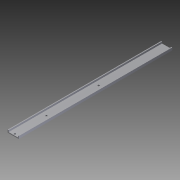
# Autodesk Inventor part: 2
Saved by Autodesk Inventor 2011 (Build 150239000, 239)
## iProperties
Created: 2011-09-24
Part Number: 2
Document SubType Name: Modeling
Designer: Matthew
Density: 1 g/cm^3
Author: Matthew
Autodesk Inventor part; units mm, degrees
ref_plane "YZ Plane" through (0, 0, 0) normal (1, 0, 0) x (0, 1, 0)
ref_plane "XZ Plane" through (0, 0, 0) normal (0, 1, 0) x (-1, 0, 0)
ref_plane "XY Plane" through (0, 0, 0) normal (0, 0, 1) x (1, 0, 0)
sketch "Sketch1" plane through (0, 0, 0) normal (0, 0, 1) x (1, 0, 0)
  line L0 (-18.7296, 9.1612) -> (16.5704, 9.1612)
  line L1 (16.5704, 9.1612) -> (16.5704, -0.3388)
  line L2 (16.5704, -0.3388) -> (-18.7296, -0.3388)
  line L3 (-18.7296, -0.3388) -> (-18.7296, 9.1612)
  line L4 (-18.7296, 4.4112) -> (16.5704, 4.4112)
  line L5 (-18.7296, 4.4112) -> (-18.7296, -0.3388)
  line L6 (-18.7296, 2.0362) -> (16.5704, 2.0362)
  line L7 (16.5704, 4.4112) -> (14.1954, 2.0362)
  line L8 (16.5704, 4.4112) -> (19.9291, 4.4112) construction
  line L9 (-18.7296, 4.4112) -> (-16.3546, 2.0362)
  line L10 (-16.3546, 2.0362) -> (-16.3546, 9.1612)
  line L11 (14.1954, 2.0362) -> (14.1954, 9.1612)
  line L12 (-16.3546, 4.4112) -> (-13.9796, 2.0362)
  line L13 (14.1954, 4.4112) -> (11.8204, 2.0362)
  line L14 (11.8204, 2.0362) -> (11.8204, 9.1612)
  line L15 (-13.9796, 2.0362) -> (-13.9796, 9.1612)
  point P0 (0, 0)
  dimension "d0" = 35.3
  dimension "d1" = 9.5
  dimension "d2" = 135
  constraints: 32 end point, 13 point on line, 8 perpendicular, 3 midpoint, 3 parallel, 2 horizontal, 1 collinear, 1 equal length
  measures "d0" distance of L1.end L2.end
  measures "d1" distance of L0.end L1.end
  measures "d2" angle of L7 L8
extrude "Extrusion1" add sketch "Sketch1" along normal blind 445 contours L0 L15 L4 L10 | L12 L6 L10 | L4 L15 L12 | L0 L11 L4 L14 | L4 L14 L6 L15 | L4 L13 L14 | L13 L11 L6
sketch "Sketch2" plane through (-13.9796, 4.4112, 0) normal (0, 1, 0) x (1, 0, 0)
  line L0 (0, -445) -> (25.8, -445) projected
  line L1 (12.9, -445) -> (12.9, -416.7)
  circle A0 centre (12.9, -416.7) radius 2.15
  line L2 (12.9, -416.7) -> (12.9, -64.7)
  circle A1 centre (12.9, -64.7) radius 2.15
  line L3 (12.9, -416.7) -> (12.9, -32.7)
  circle A2 centre (12.9, -32.7) radius 2.15
  point P0 (13.9796, 0)
  dimension "d5" = 28.3
  dimension "d6" = 4.3
  dimension "d7" = 352
  dimension "d8" = 384
  constraints: 6 end point, 3 centre point, 3 coincident, 2 collinear, 1 midpoint, 1 perpendicular
  measures "d5" distance of L1.start L1.end
  measures "d6" diameter of A0
  measures "d7" distance of L2.start L2.end
  measures "d8" distance of L2.start L3.end
extrude "Extrusion2" cut sketch "Sketch2" against normal blind 445
sketch "Sketch3" plane through (0, 0, 445) normal (0, 0, 1) x (1, 0, 0)
  line L0 (14.1954, 2.0362) -> (-16.3546, 2.0362) projected
  line L1 (14.1954, 9.1612) -> (14.1954, 2.0362) projected
  line L2 (11.8204, 9.1612) -> (14.1954, 9.1612) projected
  line L3 (11.8204, 4.4112) -> (11.8204, 9.1612) projected
  line L4 (-13.9796, 4.4112) -> (11.8204, 4.4112) projected
  line L5 (-13.9796, 9.1612) -> (-13.9796, 4.4112) projected
  line L6 (-16.3546, 9.1612) -> (-13.9796, 9.1612) projected
  line L7 (-16.3546, 2.0362) -> (-16.3546, 9.1612) projected
  point P0 (0, 0)
extrude "Extrusion3" cut sketch "Sketch3" against normal blind 419.1
sketch "Sketch4" plane through (0, 0, 0) normal (0, 0, -1) x (-1, 0, 0)
  line L0 (-14.1954, 2.0362) -> (-14.1954, 9.1612) projected
  line L1 (16.3546, 2.0362) -> (-14.1954, 2.0362) projected
  line L2 (16.3546, 9.1612) -> (16.3546, 2.0362) projected
  line L3 (13.9796, 9.1612) -> (16.3546, 9.1612) projected
  line L4 (13.9796, 4.4112) -> (13.9796, 9.1612) projected
  line L5 (-11.8204, 4.4112) -> (13.9796, 4.4112) projected
  line L6 (-11.8204, 9.1612) -> (-11.8204, 4.4112) projected
  line L7 (-14.1954, 9.1612) -> (-11.8204, 9.1612) projected
  point P0 (0, 0)
extrude "Extrusion4" add sketch "Sketch4" against normal blind 422.275
sketch "Sketch5" plane through (-16.3546, 2.0362, 0) normal (0, -1, 0) x (1, 0, 0)
  line L0 (30.55, 422.275) -> (0, 422.275) projected
  line L1 (15.275, 422.275) -> (15.275, 331.216)
  circle A0 centre (15.275, 331.216) radius 2.3495
  line L2 (15.275, 422.275) -> (15.275, 187.325)
  circle A1 centre (15.275, 187.325) radius 2.3495
  point P0 (16.3546, 0)
  dimension "d15" = 91.059
  dimension "d16" = 4.699
  dimension "d17" = 234.95
  constraints: 4 end point, 2 centre point, 2 coincident, 1 collinear, 1 midpoint, 1 perpendicular
  measures "d15" distance of L1.start L1.end
  measures "d16" diameter of A0
  measures "d17" distance of L1.start L2.end
extrude "Extrusion5" cut sketch "Sketch5" against normal blind 422.275
sketch "Sketch6" plane through (-16.3546, 2.0362, 0) normal (0, -1, 0) x (1, 0, 0)
  line L0 (30.55, 422.275) -> (0, 422.275) projected
  line L1 (15.275, 422.275) -> (15.275, 417.83)
  circle A0 centre (15.275, 417.83) radius 2.3495
  point P0 (16.3546, 0)
  dimension "d20" = 4.445
  constraints: 2 end point, 1 centre point, 1 coincident, 1 midpoint, 1 perpendicular
  measures "d20" distance of L1.start L1.end
extrude "Extrusion6" cut sketch "Sketch6" against normal blind 422.275
body "Solid1"
